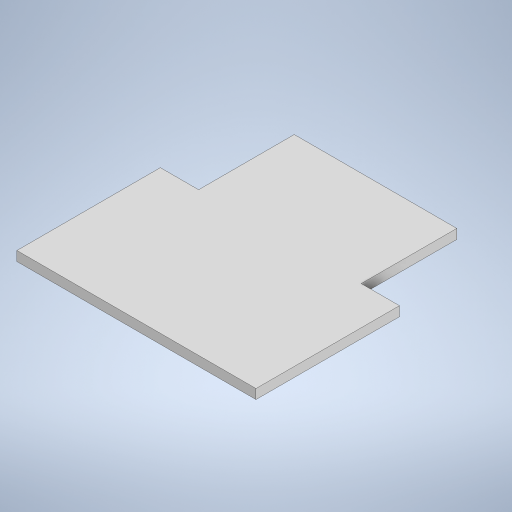
# Autodesk Inventor part: podstawa_v2
Saved by Autodesk Inventor 2023.5 (Build 275446000, 446)
## iProperties
Created: 2025-03-17
Part Number: podstawa_v2
Material: Ogólny
Document SubType Name: Modeling
Designer: kamil
Density: 1 g/cm^3
Appearance: Domyślna
Author: kamil
Autodesk Inventor part; units mm, degrees
ref_plane "YZ Plane" through (0, 0, 0) normal (1, 0, 0) x (0, 1, 0)
ref_plane "XZ Plane" through (0, 0, 0) normal (0, 1, 0) x (-1, 0, 0)
ref_plane "XY Plane" through (0, 0, 0) normal (0, 0, 1) x (1, 0, 0)
sketch "Szkic1" plane through (0, 0, 0) normal (0, 1, 0) x (-1, 0, 0)
  line L0 (0, 0) -> (-50, 0)
  line L1 (-50, 0) -> (-50, -50)
  line L2 (-50, -50) -> (0, -50)
  line L3 (0, -50) -> (0, 0)
  line L4 (0, -50) -> (-8, -50)
  line L5 (-8, -50) -> (-8, -30)
  line L6 (-8, -30) -> (0, -30)
  line L7 (0, -30) -> (0, -50)
  line L8 (-50, -50) -> (-42, -50)
  line L9 (-42, -50) -> (-42, -30)
  line L10 (-42, -30) -> (-50, -30)
  line L11 (-50, -30) -> (-50, -50)
  dimension "d0" = 50
  dimension "d1" = 50
  dimension "d2" = 8
  dimension "d3" = 20
  dimension "d4" = 8
  dimension "d5" = 20
  constraints: 24 end point, 6 parallel, 3 horizontal, 3 perpendicular, 1 coincident
  measures "d0" distance of L2.end L1.end
  measures "d1" distance of L1.end L0.end
  measures "d2" distance of L5.end L6.end
  measures "d3" distance of L4.end L5.end
  measures "d4" distance of L10.end L9.end
  measures "d5" distance of L9.end L8.end
extrude "Wyciągnięcie proste1" add sketch "Szkic1" along normal blind 2 contours L3 L6 L5 L2 L9 L10 L1 L0
